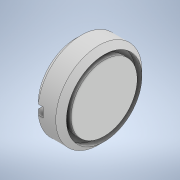
# Autodesk Inventor part: 711118
Saved by Autodesk Inventor 2022 (Build 260153000, 153)
## iProperties
Created: 2021-10-21
Part Number: 711118
Material: Типовые
Document SubType Name: Modeling
Designer: RaNSiD
Density: 1 g/cm^3
Appearance: По умолчанию
Author: RaNSiD
Autodesk Inventor part; units mm, degrees
ref_plane "YZ Plane" through (0, 0, 0) normal (1, 0, 0) x (0, 1, 0)
ref_plane "XZ Plane" through (0, 0, 0) normal (0, 1, 0) x (-1, 0, 0)
sketch "Эскиз1" plane through (0, 0, 0) normal (0, 0, 1) x (1, 0, 0)
  line L0 (0, 0) -> (0, 20)
  line L1 (0, 20) -> (2.8284, 22.8284)
  line L2 (0, 0) -> (15, 0)
  line L3 (15, 0) -> (15, 20)
  line L4 (15, 20) -> (12.1716, 22.8284)
  line L5 (12.1716, 22.8284) -> (2.8284, 22.8284)
  dimension "d0" = 20
  dimension "d1" = 4
  dimension "d2" = 135
  dimension "d3" = 15
  dimension "d4" = 4
  dimension "d5" = 135
  constraints: 12 end point, 1 horizontal, 1 parallel, 1 perpendicular, 1 vertical
  measures "d0" distance of L0.start L0.end
  measures "d1" distance of L0.end L1.end
  measures "d2" angle of L0 L1
  measures "d3" distance of L0.start L2.end
  measures "d4" distance of L3.end L4.end
  measures "d5" angle of L4 L3
revolve "Вращение1" add sketch "Эскиз1" angle 360 about axis through (0, 0, 0) along (1, 0, 0)
ref_plane "РабПлоскость1" through (0, 0, 23) normal (0, 0, 1) x (1, 0, 0)
sketch "Эскиз2" plane through (0, 0, 23) normal (0, 0, 1) x (1, 0, 0)
  line L0 (0, -20) -> (0, 20) projected
  line L1 (0, -2.5) -> (5.5, -2.5)
  line L2 (5.5, -2.5) -> (5.5, 2.5)
  line L3 (5.5, 2.5) -> (0, 2.5)
  line L4 (0, 2.5) -> (0, -2.5)
  point P0 (0, 0)
  point P1 (5.5, 0)
  point P2 (0, 0)
  point P3 (0, 2.5)
  dimension "d8" = 5
  dimension "d9" = 5.5
  constraints: 8 end point, 2 midpoint, 2 parallel, 1 horizontal, 1 horizontal alignment, 1 perpendicular, 1 point on line
  measures "d8" distance of L1.end L2.end
  measures "d9" distance of L2.end L3.end
extrude "Выдавливание1" cut sketch "Эскиз2" against normal blind 50
sketch "Эскиз3" plane through (0, 0, 0) normal (-1, 0, 0) x (0, 0, 1)
  line L0 (0, 0) -> (0, 17) construction
  dimension "d12" = 17
  constraints: 2 end point, 1 coincident, 1 vertical
  measures "d12" distance of L0.start L0.end
hole "Отверстие1" at (0, 17, 0) direction (1, 0, 0) diameter 2 depth 2 tip angle 118
sketch "Эскиз4" plane through (0, 0, 0) normal (0, 1, 0) x (-1, 0, 0)
  line L0 (-15, 20) -> (-15, -20) construction
  line L1 (-15, -20) -> (-11.5, -20)
  line L2 (-11.5, -20) -> (-11.5, -17.5)
  line L3 (-11.5, -17.5) -> (-15, -17.5)
  line L4 (-15, -17.5) -> (-15, -20)
  line L5 (-15, 0) -> (0, 0)
  line L6 (0, 1) -> (0, -1) projected
  dimension "d20" = 3.5
  dimension "d21" = 2.5
  constraints: 10 end point, 2 midpoint, 2 parallel, 1 horizontal, 1 perpendicular
  measures "d20" distance of L3.end L2.end
  measures "d21" distance of L2.end L1.end
revolve "Вращение2" cut sketch "Эскиз4" angle 360 about axis through (15, 0, 0) along (-1, 0, 0)
